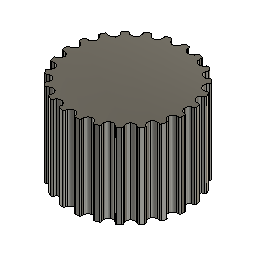
gear_23z (Autodesk Fusion 360 design; units mm, degrees)
Autodesk Fusion 360 part; units mm, degrees
sketch "Sketch1" plane through (0, 0, 0) normal (0, 0, 1) x (1, 0, 0) in component "gt2 pulley"
  circle A0 centre (0, 0) radius 7.3211 construction
  circle A1 centre (0, 0) radius 6.3171 construction
  line L0 (0, 0) -> (0, 7.3211) construction
  line L1 (0, 0) -> (0.9969, 7.2529) construction
  line L2 (0, 0) -> (1.4114, 7.1838) construction
  circle A2 centre (0, 0) radius 7.0671 construction
  arc A3 (0.3626, 6.9166) -> (0.4036, 6.6504) centre (1.3624, 6.9346) ccw
  circle A4 centre (0, 0) radius 6.9171 construction
  arc A5 (0.2171, 7.0638) -> (0, 7.0671) centre (0, 0) ccw
  arc A6 (0.3626, 6.9166) -> (0.2171, 7.0638) centre (0.2126, 6.9139) ccw
  arc A7 (0.4036, 6.6504) -> (0.8602, 6.2583) centre (0.9358, 6.8081) ccw
  arc A8 (0, 7.0671) -> (-0.2171, 7.0638) centre (0, 0) ccw
  arc A9 (-0.2171, 7.0638) -> (-0.3626, 6.9166) centre (-0.2126, 6.9139) ccw
  arc A10 (-0.4036, 6.6504) -> (-0.3626, 6.9166) centre (-1.3624, 6.9346) ccw
  arc A11 (-0.8605, 6.2582) -> (-0.4036, 6.6504) centre (-0.9358, 6.8081) ccw
  arc A12 (0.8602, 6.2583) -> (-0.8602, 6.2583) centre (0, 0) ccw
  point P0 (1.3624, 6.9346)
  point P1 (0, 7.0671)
  dimension "d18" = 14.6423
  dimension "d19" = 7.826
  dimension "d22" = 1.004
  dimension "d24" = 0.75
  dimension "d26" = 1
  dimension "d27" = 0.15
  dimension "d28" = 0.15
  dimension "d47" = 0.555
  dimension "d52" = 3.812
  constraint coincident A0.centre A1.centre
  constraint coincident A0 L0.end
  constraint vertical L0
  constraint coincident A0 L1.end
  constraint coincident A0 L2.end
  constraint concentric A1 A2
  constraint coincident A1 A7.end
  constraint coincident L1 A7.end
  constraint coincident A2 P0
  constraint coincident L2 P0
  constraint coincident P0 A3.centre
  constraint coincident A2 P1
  constraint coincident L0 P1
  constraint concentric A2 A4
  constraint coincident P1 A5.end
  constraint coincident A4 A6.centre
  constraint coincident A3.start A6.start
  constraint tangent A3 A6
  constraint tangent A3 A7
  constraint symmetric L0 A7.end A12.end
  constraint symmetric L0 A3.start A9.end
  constraint symmetric L0 A3.end A10.start
  constraint symmetric L0 A3 A10
  constraint symmetric L0 A5.start A8.end
  constraint symmetric L0 P1 A5.end
  constraint symmetric L0 A5 A8
  constraint symmetric L0 A6 A9
  constraint symmetric L0 A7 A11
  constraint coincident A1 A11.start
  constraint tangent A1 A7
  constraint coincident L1 A7.centre
  measures "d18" diameter of A0
  measures "d19" angle of L0 L1
  measures "d22" distance of A0 A1
  measures "d24" distance of A1 A2
  measures "d26" radius of A3
  measures "d27" distance of A2 A4
  measures "d28" radius of A6
  measures "d47" radius of A7
extrude "Extrude1" add sketch "Sketch1" along normal blind 10 makes body 1
pattern_circular "C-Pattern1" count 23 over 360 about axis through (0, 0, 1.75) along (0, 0, 1) of bodies 1 makes body 2 at (-1.0498, 6.2293, 3.3333) makes body 3 at (-3.364, 5.3469, 6.6667) makes body 4 at (-4.1336, 4.777, 3.3333) makes body 5 at (-5.6524, 2.8207, 6.6667) makes body 6 at (-6.2038, 1.1911, 6.6667) makes body 7 at (-6.2951, -0.5269, 6.6667) makes body 8 at (-5.9195, -2.2058, 6.6667) makes body 9 at (-5.1049, -3.721, 6.6667) makes body 10 at (-3.9117, -4.9603, 6.6667) makes body 11 at (-2.4283, -5.8317, 6.6667) makes body 12 at (-0.7649, -6.2706, 6.6667) makes body 13 at (1.5192, -6.1317, 6.6667) makes body 14 at (2.6046, -5.7552, 6.6667) makes body 15 at (3.4446, -5.2954, 3.3333) makes body 16 at (4.7455, -4.1696, 3.3333) makes body 17 at (5.6945, -2.7347, 6.6667) makes body 18 at (6.2212, -1.0969, 3.3333) makes body 19 at (6.2864, 0.6222, 6.6667) makes body 20 at (5.8854, 2.2952, 3.3333) makes body 21 at (5.0479, 3.7979, 3.3333) makes body 22 at (3.8361, 5.019, 3.3333) makes body 23 at (1.6116, 6.1081, 6.6667)
sketch "Sketch2" plane through (0, 0, 10) normal (0, 0, 1) x (-1, 0, 0)
  arc A0 (-3.9035, -5.7213) -> (-3.8558, -5.9226) centre (-3.774, -5.7969) ccw
  arc A1 (-3.8558, -5.9226) -> (-3.4847, -6.1483) centre (0, 0) ccw
  arc A2 (-3.4847, -6.1483) -> (-3.2839, -6.098) centre (-3.4107, -6.0178) ccw
  arc A3 (-3.1106, -5.892) -> (-3.2839, -6.098) centre (-2.439, -6.6329) ccw
  arc A4 (-2.5168, -5.7941) -> (-3.1106, -5.892) centre (-2.7379, -6.3032) ccw
  arc A5 (-3.9867, -4.9003) -> (-2.5168, -5.7941) centre (0, 0) ccw
  arc A6 (-3.8003, -5.4725) -> (-3.9867, -4.9003) centre (-4.3369, -5.3308) ccw
  arc A7 (-3.9035, -5.7213) -> (-3.8003, -5.4725) centre (-4.7672, -5.2171) ccw
  circle A8 centre (0, 0) radius 6.3171
  constraint concentric A1 A8
extrude "Extrude2" add sketch "Sketch2" against normal blind 10 contours A5 A8 bodies 1 2 3 4 5 6 7 8 9 10 11 12 13 14 15 16 17 18 19 20 21 22 23
extrude "Extrude4" [suppressed] in component "gt2 pulley"
pattern_circular "C-Pattern7" [suppressed] in component "gt2 pulley"
extrude "Extrude3" [suppressed] in component "gt2 pulley"
pattern_circular "C-Pattern6" [suppressed] in component "gt2 pulley"
extrude "Extrude2'" [suppressed] in component "gt2 pulley"
pattern_circular "C-Pattern5" [suppressed] in component "gt2 pulley"
extrude "Extrude1'" [suppressed] in component "gt2 pulley"
pattern_circular "C-Pattern4" [suppressed] in component "gt2 pulley"
pattern_circular "C-Pattern3" [suppressed] in component "gt2 pulley"
pattern_circular "C-Pattern2" [suppressed] in component "gt2 pulley"
pattern_circular "C-Pattern1'" [suppressed] in component "gt2 pulley"
copy_body "Body->Comp1" [suppressed] in component "Component"
copy_body "Body->Comp2" [suppressed] in component "Component'"
copy_body "Body->Comp3" [suppressed] in component "Component''"
copy_body "Body->Comp4" [suppressed] in component "Component'''"
copy_body "Body->Comp5" [suppressed] in component "Component''''"
copy_body "Body->Comp6" [suppressed] in component "Component'''''"
copy_body "Body->Comp7" [suppressed] in component "Component''''''"
copy_body "Body->Comp8" [suppressed] in component "Component'''''''"
copy_body "Body->Comp9" [suppressed] in component "Component''''''''"
copy_body "Body->Comp10" [suppressed] in component "Component'''''''''"
copy_body "Body->Comp11" [suppressed] in component "Component''''''''''"
copy_body "Body->Comp12" [suppressed] in component "Component'''''''''''"
copy_body "Body->Comp13" [suppressed] in component "Component''''''''''''"
copy_body "Body->Comp14" [suppressed] in component "Component'''''''''''''"
copy_body "Body->Comp15" [suppressed] in component "Component''''''''''''''"
copy_body "Body->Comp16" [suppressed] in component "Component'''''''''''''''"
copy_body "Body->Comp17" [suppressed] in component "Component''''''''''''''''"
copy_body "Body->Comp18" [suppressed] in component "Component'''''''''''''''''"
copy_body "Body->Comp19" [suppressed] in component "Component''''''''''''''''''"
copy_body "Body->Comp20" [suppressed] in component "Component'''''''''''''''''''"
component "gt2 pulley" placed x (1, 0, 0) y (0, 1, 0) z (0, 0, 1) at (0, 0, 0)
equation "NumTeeth = 23" comment "min 20"
equation "ToothPitch = 2 mm"
equation "PullyDia = NumTeeth * ToothPitch / PI"
equation "ToothAng = ( ( 360 / NumTeeth ) * 1 deg )"
equation "TransOffsetAngle = ToothAng * 0.2"
equation "Sholulder_Radius = 0.15 mm"
equation "Root_Radius = 0.555 mm"
equation "TransRadius = 1 mm"
equation "ToolHeight = 0.75 mm"
equation "PLD = 0.254 mm"
equation "d18 = PullyDia"
equation "d19 = ToothAng / 2"
equation "d22 = PLD + ToolHeight"
equation "d24 = ToolHeight"
equation "d26 = TransRadius"
equation "d27 = Sholulder_Radius"
equation "d31 = NumTeeth"
equation "d33 = NumTeeth"
equation "d35 = NumTeeth"
equation "d37 = NumTeeth"
equation "d41 = NumTeeth"
equation "d45 = NumTeeth"
equation "d47 = Root_Radius"
equation "d50 = NumTeeth"
